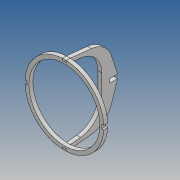
# Autodesk Inventor part: paleta expolra
Saved by Autodesk Inventor 2017 (Build 210142000, 142)
## iProperties
Part Number: paleta expolra
Material: Genérico
Document SubType Name: Modeling
Designer: Leo
Density: 1 g/cm^3
Appearance: Valor por defecto
Author: Leo
Autodesk Inventor part; units mm, degrees
ref_plane "YZ Plane" through (0, 0, 0) normal (1, 0, 0) x (0, 1, 0)
ref_plane "XZ Plane" through (0, 0, 0) normal (0, 1, 0) x (-1, 0, 0)
ref_plane "XY Plane" through (0, 0, 0) normal (0, 0, 1) x (1, 0, 0)
sketch "Boceto1" plane through (0, 0, 0) normal (0, 1, 0) x (-1, 0, 0)
  circle A0 centre (0, 0) radius 45
  line L0 (49.9375, 2.5) -> (47.5, 2.5)
  line L1 (47.5, 2.5) -> (47.5, -2.5)
  line L2 (47.5, -2.5) -> (49.9375, -2.5)
  line L3 (-2.5, 49.9375) -> (-2.5, 47.5)
  line L4 (-2.5, 47.5) -> (2.5, 47.5)
  line L5 (2.5, 47.5) -> (2.5, 49.9375)
  line L6 (-49.9375, -2.5) -> (-47.5, -2.5)
  line L7 (-47.5, -2.5) -> (-47.5, 2.5)
  line L8 (-47.5, 2.5) -> (-49.9375, 2.5)
  line L9 (2.5, -49.9375) -> (2.5, -47.5)
  line L10 (2.5, -47.5) -> (-2.5, -47.5)
  line L11 (-2.5, -47.5) -> (-2.5, -49.9375)
  arc A1 (49.9375, 2.5) -> (2.5, 49.9375) centre (0, 0) ccw
  arc A2 (-2.5, 49.9375) -> (-49.9375, 2.5) centre (0, 0) ccw
  arc A3 (-49.9375, -2.5) -> (-2.5, -49.9375) centre (0, 0) ccw
  arc A4 (2.5, -49.9375) -> (49.9375, -2.5) centre (0, 0) ccw
  point P0 (47.5, 0)
  point P1 (0, 47.5)
  point P2 (-47.5, 0)
  point P3 (0, -47.5)
  dimension "di" = 90
  dimension "d2" = 2.5
  dimension "esp" = 5
  dimension "d6" = 360
  dimension "d8" = 5
  constraints: 24 end point, 8 point on circle, 5 centre point, 2 coincident, 2 perpendicular, 1 horizontal, 1 horizontal alignment, 1 midpoint, 33 other
  measures "di" diameter of A0
  measures "d2" distance edge to line of A0 L1
  measures "esp" distance between parallel lines of L2 L0
  measures "d8" radial gap between concentric circles of A0 A1
extrude "Extrusión1" add sketch "Boceto1" against normal blind 5
sketch "Boceto2" plane through (0, 0, 0) normal (1, 0, 0) x (0, 1, 0)
  line L0 (-5, 47.5) -> (-5, 49.9375) projected
  line L1 (0, 49.9375) -> (-5, 49.9375) projected
  line L2 (-5, -49.9375) -> (-5, -47.5) projected
  line L3 (0, -49.9375) -> (-5, -49.9375) projected
  line L4 (0, -47.5) -> (-5, -47.5) projected
  line L5 (0, 47.5) -> (-5, 47.5) projected
  line L6 (0, 47.5) -> (0, 45)
  line L7 (0, -47.5) -> (0, -45)
  line L8 (0, -45) -> (13.1359, -43.6194)
  arc A0 (13.1359, -43.6194) -> (40, -13.7837) centre (10, -13.7837) ccw
  line L9 (40, -13.7837) -> (40, 13.7837)
  arc A1 (40, 13.7837) -> (13.1359, 43.6194) centre (10, 13.7837) ccw
  line L10 (13.1359, 43.6194) -> (0, 45)
  line L11 (0, 49.9375) -> (26.7876, 47.122)
  arc A2 (52.1835, 26.5568) -> (26.7876, 47.122) centre (23.6518, 17.2863) ccw
  line L12 (52.1835, 26.5568) -> (60, 2.5)
  line L13 (60, 2.5) -> (50, 2.5)
  line L14 (50, 2.5) -> (50, -2.5)
  line L15 (50, -2.5) -> (60, -2.5)
  line L16 (60, -2.5) -> (52.1835, -26.5568)
  arc A3 (26.7876, -47.122) -> (52.1835, -26.5568) centre (23.6518, -17.2863) ccw
  line L17 (26.7876, -47.122) -> (0, -49.9375)
  point P0 (0, 0)
  point P1 (40, 0)
  point P2 (50, 0)
  dimension "d11" = 12
  dimension "d12" = 40
  dimension "d13" = 90
  dimension "d14" = 5
  dimension "d15" = 20
  dimension "d16" = 10
  dimension "d17" = 18
  dimension "d18" = 30
  constraints: 24 end point, 8 point on circle, 6 tangent, 5 equal length, 4 centre point, 3 equal radius, 3 vertical, 2 horizontal alignment, 2 midpoint, 2 parallel, 2 perpendicular, 1 horizontal
  measures "d11" angle of L8 L10
  measures "d12" distance from line of L9 point (0, 0)
  measures "d13" distance of L7.end L6.end
  measures "d14" distance of L13.end L14.end
  measures "d15" distance from line of L15.end L9
  measures "d16" distance of L14.end L15.end
  measures "d17" angle of L12 L9
  measures "d18" radius of A1
extrude "Extrusión2" add sketch "Boceto2" along normal mid plane 5 separate body
equation "\"d2\" = 0.5 * d0"
equation "\"d8\" = d0"
equation "\"d9\" = esp"
equation "\"d13\" = di"
equation "\"d14\" = esp"
equation "\"d15\" = 0.5 * d12"
equation "\"d16\" = 0.5 * d15"
equation "\"d18\" = 0.333333 * d13"
equation "\"d19\" = esp"
equation "\"d0\" = 5"
